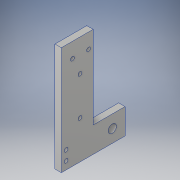
# Autodesk Inventor part: PaddleCollection2.1ServoSupport
Saved by Autodesk Inventor 2019 (Build 230136000, 136)
## iProperties
Created: 2018-10-23
Part Number: PaddleCollection2.1ServoSupport
Material: Aluminum 6061
Document SubType Name: Modeling
Designer: User
Density: 2.7 g/cm^3
Appearance: Aluminum - Flat
Author: User
Autodesk Inventor part; units mm, degrees
ref_plane "YZ Plane" through (0, 0, 0) normal (1, 0, 0) x (0, 1, 0)
ref_plane "XZ Plane" through (0, 0, 0) normal (0, 1, 0) x (-1, 0, 0)
ref_plane "XY Plane" through (0, 0, 0) normal (0, 0, 1) x (1, 0, 0)
sketch "Sketch1" plane through (0, 0, 0) normal (1, 0, 0) x (0, 1, 0)
  line L0 (0, 0) -> (107.95, 0)
  line L1 (107.95, 0) -> (107.95, -57.15)
  line L2 (107.95, -57.15) -> (0, -57.15)
  line L3 (0, -57.15) -> (0, 0)
  line L4 (107.95, -57.15) -> (25.4, -57.15)
  line L5 (25.4, -57.15) -> (25.4, -25.4)
  line L6 (25.4, -25.4) -> (107.95, -25.4)
  line L7 (107.95, -25.4) -> (107.95, -57.15)
  dimension "d0" = 107.95
  dimension "d1" = 57.15
  dimension "d2" = 82.55
  dimension "d3" = 31.75
  constraints: 16 end point, 4 parallel, 2 horizontal, 2 perpendicular
  measures "d0" distance of L1.end L2.end
  measures "d1" distance of L0.end L1.end
  measures "d2" distance of L5.end L6.end
  measures "d3" distance of L4.end L5.end
extrude "Extrusion1" add sketch "Sketch1" along normal blind 6.35 contours L0 L1 L6 L5 L2 L3
sketch "Sketch2" plane through (6.35, 0, 0) normal (1, 0, 0) x (0, 0, -1)
  line L0 (0, 0) -> (57.15, 0) projected
  line L1 (57.15, 25.4) -> (25.4, 25.4) projected
  line L2 (25.4, 25.4) -> (25.4, 107.95) projected
  line L3 (25.4, 107.95) -> (0, 107.95) projected
  line L4 (0, 107.95) -> (0, 0) projected
  line L5 (0, 0) -> (57.15, 0) projected
  line L6 (57.15, 0) -> (57.15, 25.4) projected
  point P0 (4.699, 92.9894)
  point P1 (20.701, 92.9894)
  dimension "d6" = 92.9894
  dimension "d7" = 92.9894
  dimension "d8" = 16.002
  dimension "d9" = 25.4
  dimension "d10" = 4.699
  measures "d6" distance from line of L0 point (4.699, 92.989)
  measures "d7" distance from line of L0 point (20.701, 92.989)
  measures "d8" distance of point (20.701, 92.989) point (4.699, 92.989)
  measures "d9" distance of L2.end L3.end
  measures "d10" distance from line of L4 point (4.699, 92.989)
hole "Hole1" at (6.35, 92.9894, -4.699) at (6.35, 92.9894, -20.701) direction (-1, 0, 0) diameter 3.81 end through all
sketch "Sketch3" plane through (6.35, 0, 0) normal (1, 0, 0) x (0, 0, -1)
  line L0 (57.15, 25.4) -> (25.4, 25.4) projected
  line L1 (57.15, 0) -> (57.15, 25.4) projected
  point P0 (0, 0)
  point P1 (44.45, 12.7)
  dimension "d18" = 12.7
  dimension "d19" = 12.7
  measures "d18" distance from line of L0 point (44.45, 12.7)
  measures "d19" distance from line of L1 point (44.45, 12.7)
hole "Hole2" at (6.35, 12.7, -44.45) direction (-1, 0, 0) diameter 8.128 end through all
sketch "Sketch4" plane through (6.35, 0, 0) normal (1, 0, 0) x (0, 0, -1)
  line L0 (0, 107.95) -> (0, 0) projected
  line L1 (0, 0) -> (57.15, 0) projected
  line L2 (25.4, 25.4) -> (25.4, 107.95) projected
  point P0 (12.1412, 76.2)
  point P1 (12.1412, 38.1)
  dimension "d29" = 38.1
  dimension "d30" = 76.2
  dimension "d38" = 13.2588
  dimension "d39" = 13.2588
  measures "d29" distance from line of L1 point (12.141, 38.1)
  measures "d30" distance from line of L1 point (12.141, 76.2)
  measures "d38" distance from line of L2 point (12.141, 76.2)
  measures "d39" distance from line of L2 point (12.141, 38.1)
hole "Hole3" at (6.35, 76.2, -12.1412) at (6.35, 38.1, -12.1412) direction (-1, 0, 0) diameter 3.81 depth 10.9728 tip angle 118
sketch "Sketch5" plane through (0, 0, 0) normal (0, 0, 1) x (1, 0, 0)
  line L0 (0, 107.95) -> (0, 0) projected
  line L1 (0, 0) -> (6.35, 0) projected
  line L2 (6.35, 107.95) -> (6.35, 0) projected
  line L3 (0, 107.95) -> (6.35, 107.95) projected
extrude "Extrusion2" add sketch "Sketch5" along normal blind 6.35
sketch "Sketch6" plane through (6.35, 0, 0) normal (1, 0, 0) x (0, 0, -1)
  line L0 (-6.35, 0) -> (-6.35, 107.95) projected
  line L1 (57.15, 0) -> (-6.35, 0) projected
  point P0 (0, 0)
  point P1 (-1.5875, 17.4625)
  point P2 (-1.5875, 7.9375)
  dimension "d42" = 4.7625
  dimension "d43" = 4.7625
  dimension "d44" = 9.525
  dimension "d45" = 7.9375
  measures "d42" distance from line of L0 point (-1.587, 17.462)
  measures "d43" distance from line of L0 point (-1.588, 7.938)
  measures "d44" distance of point (-1.587, 17.462) point (-1.588, 7.938)
  measures "d45" distance from line of L1 point (-1.588, 7.938)
hole "Hole4" at (6.35, 17.4625, 1.5875) at (6.35, 7.9375, 1.5875) direction (-1, 0, 0) diameter 3.81 end through all
equation "\"d7\" = d6"
equation "\"d10\" = -0.5 * d8 + 0.5 * d9"
equation "\"d39\" = d38"
equation "\"d43\" = d42"
body "Solid1"
